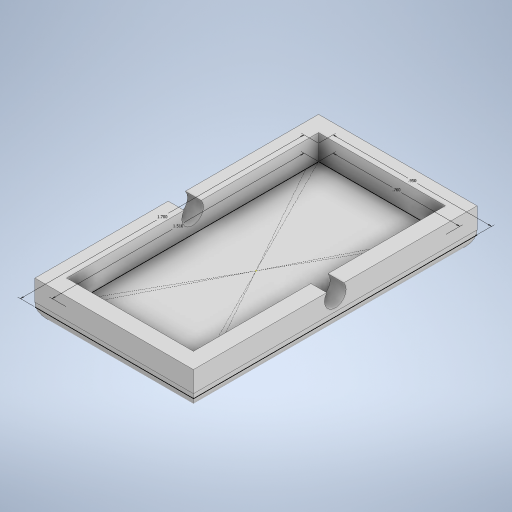
# Autodesk Inventor part: HomemadeSensorHousing 8020-Lid
Saved by Autodesk Inventor 2024.1 (Build 281209000, 209)
## iProperties
Created: 2024-07-23
Part Number: HomemadeSensorHousing 8020-Lid
Material: Generic
Document SubType Name: Modeling
Designer: pab2
Density: 1 g/cm^3
Appearance: Default
Author: pab2
Autodesk Inventor part; units mm, degrees
ref_plane "YZ Plane" through (0, 0, 0) normal (1, 0, 0) x (0, 1, 0)
ref_plane "XZ Plane" through (0, 0, 0) normal (0, 1, 0) x (-1, 0, 0)
ref_plane "XY Plane" through (0, 0, 0) normal (0, 0, 1) x (1, 0, 0)
sketch "Sketch1" plane through (0, 0, 0) normal (0, 1, 0) x (-1, 0, 0)
  line L0 (-12.065, 21.59) -> (12.065, 21.59)
  line L1 (12.065, 21.59) -> (12.065, -21.59)
  line L2 (12.065, -21.59) -> (-12.065, -21.59)
  line L3 (-12.065, -21.59) -> (-12.065, 21.59)
  line L4 (-12.065, 21.59) -> (12.065, -21.59) construction
  line L5 (12.065, 21.59) -> (-12.065, -21.59) construction
  line L6 (-9.652, 19.177) -> (9.652, 19.177)
  line L7 (9.652, 19.177) -> (9.652, -19.177)
  line L8 (9.652, -19.177) -> (-9.652, -19.177)
  line L9 (-9.652, -19.177) -> (-9.652, 19.177)
  line L10 (-9.652, 19.177) -> (9.652, -19.177) construction
  line L11 (9.652, 19.177) -> (-9.652, -19.177) construction
  point P0 (0, 0)
  dimension "d0" = 24.13
  dimension "d1" = 43.18
  dimension "d2" = 19.304
  dimension "d3" = 38.354
  constraints: 24 end point, 4 midpoint, 4 parallel, 2 horizontal, 2 perpendicular
  measures "d0" distance of L1.end L2.end
  measures "d1" distance of L0.end L1.end
  measures "d2" distance of L7.end L8.end
  measures "d3" distance of L6.end L7.end
extrude "Extrusion1" add sketch "Sketch1" along normal blind 3.81
extrude "Extrusion2" add sketch "Sketch1" against normal blind 2.54 contours L0 L1 L2 L3 | L6 L7 L8 L9
sketch "Sketch2" plane through (-9.652, 3.81, 19.177) normal (1, 0, 0) x (0, 0, -1)
  line L0 (19.177, -3.81) -> (19.177, -1.016)
  dimension "d8" = 2.794
  constraints: 2 end point, 1 vertical
  measures "d8" distance of L0.start L0.end
hole "Hole1" at (-9.652, 2.794, 0) direction (-1, 0, 0) diameter 3.302 end through all both
fillet "Fillet1" radius 3.175 4 edges at (0, -2.54, -21.59) (12.065, -2.54, 0) (-12.065, -2.54, 0) (0, -2.54, 21.59)
body "Solid1"
